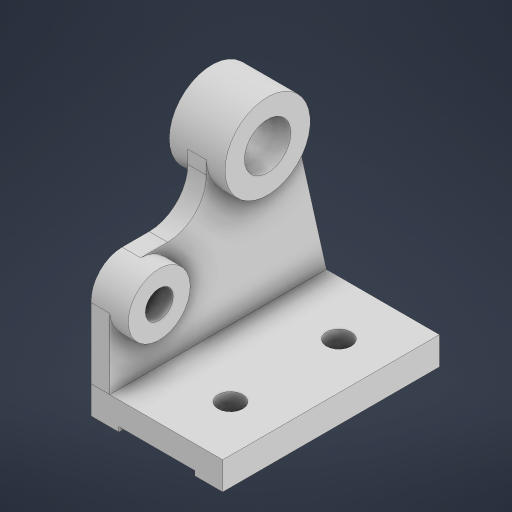
# Autodesk Inventor part: Część12
Saved by Autodesk Inventor 2023 (Build 270158000, 158)
## iProperties
Created: 2023-05-07
Part Number: Część12
Material: Ogólny
Document SubType Name: Modeling
Designer: Adam
Density: 1 g/cm^3
Appearance: Domyślna
Author: Adam
Autodesk Inventor part; units mm, degrees
ref_plane "YZ Plane" through (0, 0, 0) normal (1, 0, 0) x (0, 1, 0)
ref_plane "XZ Plane" through (0, 0, 0) normal (0, 1, 0) x (-1, 0, 0)
ref_plane "XY Plane" through (0, 0, 0) normal (0, 0, 1) x (1, 0, 0)
sketch "Szkic1" plane through (0, 0, 0) normal (0, 1, 0) x (-1, 0, 0)
  line L0 (0, 0) -> (-85, 0)
  line L1 (-85, 0) -> (-85, 140)
  line L2 (-85, 140) -> (0, 140)
  line L3 (0, 140) -> (0, 0)
  dimension "d0" = 85
  dimension "d1" = 140
  constraints: 8 end point, 2 parallel, 1 coincident, 1 horizontal, 1 perpendicular
  measures "d0" distance of L1.end L2.end
  measures "d1" distance of L0.end L1.end
sketch "Szkic2" plane through (0, 0, 0) normal (1, 0, 0) x (0, 1, 0)
  circle A0 centre (46.4724, 120) radius 20
  line L0 (47.5406, 139.9715) -> (0, 139.9715)
  circle A1 centre (100, 50) radius 27.5
  line L1 (0, 0) -> (100, 22.5)
  line L2 (100, 77.5) -> (91.4724, 77.5)
  line L3 (66.4724, 102.5) -> (66.4724, 120)
  arc A2 (66.4724, 102.5) -> (91.4724, 77.5) centre (91.4724, 102.5) ccw
  line L4 (0, 0) -> (0, 139.9715)
  point P0 (45.4042, 139.9715)
  dimension "d2" = 40
  dimension "d3" = 120
  dimension "d4" = 55
  dimension "d5" = 100
  dimension "d6" = 50
  dimension "d7" = 25
  constraints: 10 end point, 6 point on circle, 3 centre point, 3 tangent, 2 horizontal, 1 vertical
  measures "d2" diameter of A0
  measures "d3" vertical distance of L1.start A0.centre
  measures "d4" diameter of A1
  measures "d5" horizontal distance of L1.start A1.centre
  measures "d6" vertical distance of L1.start A1.centre
  measures "d7" radius of A2
extrude "Wyciągnięcie proste1" add sketch "Szkic2" along normal blind 12 contours L3 A2 L2 A1 L1 L4 L0 A0
extrude "Wyciągnięcie proste2" add sketch "Szkic1" against normal blind 18
sketch "Szkic3" plane through (0, 0, 0) normal (-1, 0, 0) x (0, 0, 1)
  arc A0 (22.5, 100) -> (77.5, 100) centre (50, 100) ccw projected
  circle A1 centre (50, 100) radius 27.5
  point P0 (0, 0)
  constraints: 1 centre point, 1 coincident
extrude "Wyciągnięcie proste3" add sketch "Szkic3" along normal blind 12 and the other way blind 24
sketch "Szkic4" plane through (0, 0, 0) normal (-1, 0, 0) x (0, 0, 1)
  arc A0 (120, 66.4724) -> (139.9715, 45.4042) centre (120, 46.4724) ccw projected
  circle A1 centre (120, 46.4724) radius 20
  point P0 (0, 0)
  point P1 (139.9715, 45.4042)
  constraints: 1 centre point, 1 coincident
extrude "Wyciągnięcie proste4" add sketch "Szkic4" against normal blind 24
sketch "Szkic5" plane through (24, 100, 50) normal (1, 0, 0) x (0, 0, -1)
  point P0 (50, -100)
  point P1 (0, 0)
hole "Otwór1" at (24, 100, 50) direction (-1, 0, 0) diameter 30 end through all
sketch "Szkic6" plane through (24, 46.4724, 120) normal (1, 0, 0) x (0, 0, -1)
  point P0 (120, -46.4724)
  point P1 (0, 0)
hole "Otwór2" at (24, 46.4724, 120) direction (-1, 0, 0) diameter 18 end through all
sketch "Szkic7" plane through (0, 0, 0) normal (0, 1, 0) x (1, 0, 0)
  line L0 (0, -140) -> (85, -140) projected
  line L1 (85, -140) -> (85, 0) projected
  point P0 (0, 0)
  point P1 (55, -105)
  point P2 (55, -35)
  dimension "d32" = 35
  dimension "d33" = 70
  dimension "d34" = 30
  dimension "d35" = 30
  measures "d32" distance from line of point (55, -105) L0
  measures "d33" distance of point (55, -35) point (55, -105)
  measures "d34" distance from line of L1 point (55, -105)
  measures "d35" distance from line of L1 point (55, -35)
hole "Otwór3" at (55, 0, 105) at (55, 0, 35) direction (0, -1, 0) diameter 16 end through all
sketch "Szkic8" plane through (0, -18, 0) normal (0, -1, 0) x (1, 0, 0)
  line L0 (0, 0) -> (85, 0) projected
  line L1 (18, 140) -> (67, 140)
  line L2 (67, 140) -> (67, 0)
  line L3 (67, 0) -> (18, 0)
  line L4 (18, 0) -> (18, 140)
  line L5 (0, 140) -> (0, 0) projected
  line L6 (85, 0) -> (85, 140) projected
  point P0 (18, 0)
  dimension "d43" = 18
  dimension "d44" = 18
  constraints: 8 end point, 2 parallel, 1 horizontal, 1 perpendicular, 1 point on line
  measures "d43" distance between parallel lines of L4 L5
  measures "d44" distance between parallel lines of L6 L2
extrude "Wyciągnięcie proste5" cut sketch "Szkic8" against normal blind 3
